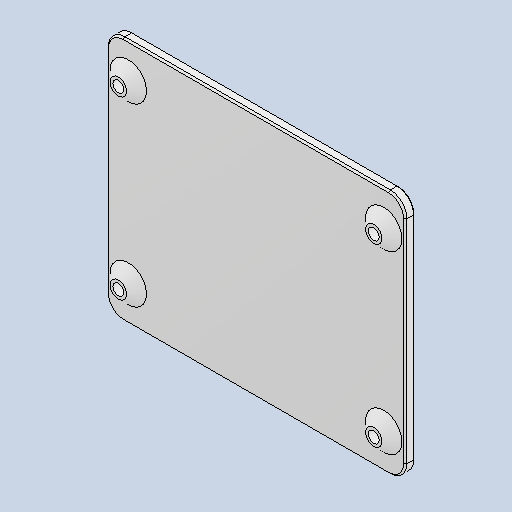
# Autodesk Inventor part: temp-logger-base-plate
Saved by Autodesk Inventor 2026 (Build 300175050, 175E)
## iProperties
Created: 2025-07-16
Part Number: temp-logger-base-plate
Material: ABS Plastic
Document SubType Name: Modeling
Designer: kuzmin
Density: 1.06 g/cm^3
Appearance: Smooth - White
Author: kuzmin
Autodesk Inventor part; units mm, degrees
ref_plane "YZ Plane" through (0, 0, 0) normal (1, 0, 0) x (0, 1, 0)
ref_plane "XZ Plane" through (0, 0, 0) normal (0, 1, 0) x (-1, 0, 0)
ref_plane "XY Plane" through (0, 0, 0) normal (0, 0, 1) x (1, 0, 0)
sketch "Sketch1" plane through (0, 0, 0) normal (0, 0, 1) x (1, 0, 0)
  line L0 (-45, 37) -> (45, 37)
  line L1 (45, 37) -> (45, -37)
  line L2 (45, -37) -> (-45, -37)
  line L3 (-45, -37) -> (-45, 37)
  line L4 (-38.5, 26.5) -> (38.5, 26.5) construction
  line L5 (38.5, 26.5) -> (38.5, -26.5) construction
  line L6 (38.5, -26.5) -> (-38.5, -26.5) construction
  line L7 (-38.5, -26.5) -> (-38.5, 26.5) construction
  circle A0 centre (-38.5, 26.5) radius 2.5
  circle A1 centre (38.5, 26.5) radius 2.5
  circle A2 centre (38.5, -26.5) radius 2.5
  circle A3 centre (-38.5, -26.5) radius 2.5
  point P0 (0, 0)
  point P1 (45, 0)
  point P2 (0, 37)
  point P3 (38.5, 0)
  point P4 (0, 26.5)
  dimension "d0" = 90
  dimension "d1" = 74
  dimension "d2" = 77
  dimension "d3" = 53
  dimension "d14" = 5
  constraints: 16 end point, 8 coincident, 4 centre point, 4 midpoint, 4 parallel, 3 equal radius, 2 horizontal, 2 horizontal alignment, 2 perpendicular, 2 vertical alignment
  measures "d0" distance of L0.start L0.end
  measures "d1" distance of L0.end L1.end
  measures "d2" distance of L4.start L4.end
  measures "d3" distance of L4.end L5.end
  measures "d14" diameter of A0
extrude "Extrusion1" add sketch "Sketch1" along normal blind 3 contours L0 L1 L2 L3 | A0 | A1 | A2 | A3
extrude "Extrusion2" add sketch "Sketch1" along normal blind 6 contours A0 | A1 | A2 | A3
chamfer "Chamfer1" distance 3 angle 45 4 edges at (-41, 26.5, 3) (36, 26.5, 3) (36, -26.5, 3) (-41, -26.5, 3)
hole "Hole1" at (38.5, 26.5, 0) at (38.5, -26.5, 0) at (-38.5, -26.5, 0) at (-38.5, 26.5, 0) direction (0, 0, 1) diameter 3.3 end through all
fillet "Fillet1" radius 5 4 edges at (45, 37, 1.5) (45, -37, 1.5) (-45, -37, 1.5) (-45, 37, 1.5)
chamfer "Chamfer2" distance 0.5 angle 45 9 edges at (0, 37, 0) (-43.5355, 35.5355, 0) (-45, 0, 0) (-43.5355, -35.5355, 0) (0, -37, 0) (43.5355, -35.5355, 0) (45, 0, 0) (43.5355, 35.5355, 0) (0, 37, 3)
equation "\"d0\" = length"
equation "\"d1\" = width"
equation "\"d4\" = thickness"
equation "\"d15\" = thickness + bump"
equation "\"width\" = 74"
equation "\"length\" = 90"
equation "\"thickness\" = 3"
equation "\"bump\" = 3"
body "Solid1"
